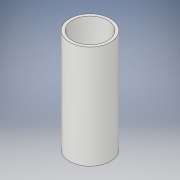
# Autodesk Inventor part: PVC Pipe 2 IN D 6 IN L
Saved by Autodesk Inventor 2019 (Build 230136000, 136)
## iProperties
Created: 2019-07-06
Part Number: PVC Pipe 2 IN D 6 IN L
Material: PVC-Piping
Document SubType Name: Modeling
Designer: J. LENDI
Mass: 155.92 g
Surface Area: 552.617 cm^2
Volume: 111.372 cm^3
Density: 1.4 g/cm^3
Appearance: Smooth - White
Author: J. LENDI
Autodesk Inventor part; units mm, degrees
ref_plane "YZ Plane" through (0, 0, 0) normal (1, 0, 0) x (0, 1, 0)
ref_plane "XZ Plane" through (0, 0, 0) normal (0, 1, 0) x (-1, 0, 0)
ref_plane "XY Plane" through (0, 0, 0) normal (0, 0, 1) x (1, 0, 0)
sketch "Sketch1" plane through (0, 0, 0) normal (0, 1, 0) x (-1, 0, 0)
  circle A0 centre (0, 0) radius 30.1625
  circle A1 centre (0, 0) radius 26.0223
  dimension "d0" = 60.325
  dimension "d1" = 52.0446
  constraints: 2 centre point, 2 coincident
  measures "d0" diameter of A0
  measures "d1" diameter of A1
extrude "Extrusion1" add sketch "Sketch1" along normal mid plane 152.4
body "Solid1"
